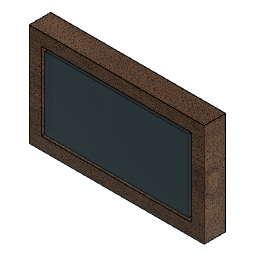
Glowing Square (Autodesk Fusion 360 design; units mm, degrees)
Autodesk Fusion 360 part; units mm, degrees
sketch "Sketch2" plane through (0, 0, 0) normal (0, 1, 0) x (1, 0, 0)
  line L0 (0, 0) -> (256, 0)
  line L1 (256, 0) -> (256, 128)
  line L2 (256, 128) -> (0, 128)
  line L3 (0, 128) -> (0, 0)
  dimension "d1" = 256
  dimension "d2" = 128
  constraint horizontal L0
  constraint vertical L1
  constraint horizontal L2
  constraint vertical L3
  constraint coincident L0.start L3.end
  measures "d1" distance of L0.start L0.end
  measures "d2" distance of L0.start L2.end
extrude "Extrude1" add sketch "Sketch2" along normal blind 14 makes body 1
chamfer "Chamfer1" distance 1 distance2 14 4 edges at (128, 14, 0) (256, 14, -64) (0, 14, -64) (128, 14, -128) measured on face at (85.3333, 14, -85.3333) measured on face at (85.3333, 14, -85.3333) measured on face at (85.3333, 14, -85.3333) measured on face at (85.3333, 14, -85.3333) on bodies 1
sketch "Sketch3" plane through (0, 14, 0) normal (0, 1, 0) x (-1, 0, 0)
  line L0 (-255, -127) -> (-1, -127)
  line L1 (-1, -127) -> (-1, -1)
  line L2 (-1, -1) -> (-255, -1)
  line L3 (-255, -1) -> (-255, -127)
  circle A0 centre (-248, -8) radius 1.5
  circle A1 centre (-128, -8) radius 1.5
  circle A2 centre (-8, -8) radius 1.5
  circle A3 centre (-248, -120) radius 1.5
  circle A4 centre (-128, -120) radius 1.5
  circle A5 centre (-8, -120) radius 1.5
  dimension "d7" = 3
  dimension "d8" = 7
  dimension "d9" = 7
  dimension "d10" = 3
  dimension "d11" = 127
  dimension "d12" = 3
  dimension "d13" = 7
  dimension "d14" = 3
  dimension "d15" = 7
  dimension "d16" = 3
  dimension "d17" = 3
  measures "d7" diameter of A0
  measures "d8" distance of L3 A0.centre
  measures "d9" distance of L2 A0.centre
  measures "d10" diameter of A1
  measures "d11" distance of L3 A1.centre
  measures "d12" diameter of A2
  measures "d13" distance of L1 A2.centre
  measures "d14" diameter of A3
  measures "d15" distance of L0 A3.centre
  measures "d16" diameter of A4
  measures "d17" diameter of A5
extrude "Extrude2" cut sketch "Sketch3" against normal blind 10 contours A0 | A1 | A2 | A3 | A4 | A5 bodies 1
sketch "Sketch4" plane through (0, 14, 0) normal (0, 1, 0) x (-1, 0, 0)
  circle A0 centre (-8, -120) radius 1.5
  circle A1 centre (-248, -8) radius 1.5
  circle A2 centre (-128, -120) radius 1.5
  circle A3 centre (-8, -8) radius 1.5
  circle A4 centre (-128, -8) radius 1.5
  circle A5 centre (-248, -120) radius 1.5
  line L0 (-255, -127) -> (-1, -127)
  line L1 (-1, -127) -> (-1, -1)
  line L2 (-1, -1) -> (-255, -1)
  line L3 (-255, -1) -> (-255, -127)
  line L4 (-103, -24) -> (-43, -24)
  line L5 (-43, -24) -> (-43, -104)
  line L6 (-43, -104) -> (-103, -104)
  line L7 (-103, -104) -> (-103, -24)
  dimension "d20" = 60
  dimension "d21" = 80
  dimension "d22" = 42
  dimension "d23" = 23
  constraint horizontal L4
  constraint vertical L5
  constraint horizontal L6
  constraint vertical L7
  measures "d20" distance of L4.start L4.end
  measures "d21" distance of L4.start L6.end
  measures "d22" distance of L1 L5
  measures "d23" distance of L0 L6
extrude "Extrude3" add sketch "Sketch4" along normal blind 20 contours L4 L5 L6 L7 bodies 1
sketch "Sketch5" plane through (0, 0, 0) normal (0, -1, 0) x (1, 0, 0)
  line L0 (0, 0) -> (0, -128)
  line L1 (0, -128) -> (256, -128)
  line L2 (256, -128) -> (256, 0)
  line L3 (256, 0) -> (0, 0)
copy_body "CutPasteBodies1" bodies 1 removing the originals makes body 2 in component "Display"
sketch "Sketch1" plane through (0, 14, 0) normal (0, 1, 0) x (-1, 0, 0) in component "Display"
  line L0 (-103, -104) -> (-103, -24)
  line L1 (-103, -24) -> (-43, -24)
  line L2 (-43, -24) -> (-43, -104)
  line L3 (-43, -104) -> (-103, -104)
  circle A0 centre (-8, -120) radius 1.5
  circle A1 centre (-248, -8) radius 1.5
  circle A2 centre (-128, -120) radius 1.5
  circle A3 centre (-8, -8) radius 1.5
  circle A4 centre (-128, -8) radius 1.5
  circle A5 centre (-248, -120) radius 1.5
  line L4 (-255, -127) -> (-1, -127)
  line L5 (-1, -127) -> (-1, -1)
  line L6 (-1, -1) -> (-255, -1)
  line L7 (-255, -1) -> (-255, -127)
sketch "Sketch1 (2)" plane through (0, 0, 0) normal (0, 1, 0) x (1, 0, 0) in component "Frame"
  line L0 (-27, -27) -> (283, -27)
  line L1 (283, -27) -> (283, 155)
  line L2 (283, 155) -> (-27, 155)
  line L3 (-27, 155) -> (-27, -27)
  line L4 (-5, -5) -> (261, -5)
  line L5 (261, -5) -> (261, 133)
  line L6 (261, 133) -> (-5, 133)
  line L7 (-5, 133) -> (-5, -5)
  dimension "d26" = 310
  dimension "d27" = 182
  dimension "d28" = 27
  dimension "d29" = 27
  dimension "d30" = 22
  dimension "d31" = 22
  dimension "d32" = 22
  dimension "d33" = 22
  constraint horizontal L0
  constraint vertical L1
  constraint horizontal L2
  constraint vertical L3
  constraint horizontal L4
  constraint vertical L5
  constraint horizontal L6
  constraint vertical L7
  measures "d26" distance of L0.start L0.end
  measures "d27" distance of L0.start L2.end
  measures "d28" distance of origin L3
  measures "d29" distance of L0 origin
  measures "d30" distance of L3 L7
  measures "d31" distance of L1 L5
  measures "d32" distance of L0 L4
  measures "d33" distance of L2 L6
extrude "Extrude1'" add sketch "Sketch1 (2)" along normal blind 38 separate body makes body 3 in component "Frame"
sketch "Sketch1 (3)" plane through (0, 14, 0) normal (0, 1, 0) x (-1, 0, 0) in component "Display Mount"
  line L0 (-103, -104) -> (-103, -24)
  line L1 (-103, -24) -> (-43, -24)
  line L2 (-43, -24) -> (-43, -104)
  line L3 (-43, -104) -> (-103, -104)
  circle A0 centre (-8, -120) radius 1.5
  circle A1 centre (-248, -8) radius 1.5
  circle A2 centre (-128, -120) radius 1.5
  circle A3 centre (-8, -8) radius 1.5
  circle A4 centre (-128, -8) radius 1.5
  circle A5 centre (-248, -120) radius 1.5
  line L4 (-255, -127) -> (-1, -127)
  line L5 (-1, -127) -> (-1, -1)
  line L6 (-1, -1) -> (-255, -1)
  line L7 (-255, -1) -> (-255, -127)
  line L8 (-261, 5) -> (5, 5)
  line L9 (5, 5) -> (5, -133)
  line L10 (5, -133) -> (-261, -133)
  line L11 (-261, -133) -> (-261, 5)
  line L12 (-256, -128) -> (-256, 0)
  line L13 (-256, 0) -> (0, 0)
  line L14 (-243, -13) -> (-13, -13)
  line L15 (-13, -13) -> (-13, -115)
  line L16 (-13, -115) -> (-243, -115)
  line L17 (-243, -115) -> (-243, -13)
  dimension "d36" = 266
  dimension "d37" = 138
  dimension "d38" = 5
  dimension "d39" = 5
  dimension "d40" = 5
  dimension "d41" = 5
  dimension "d42" = 5
  dimension "d43" = 5
  constraint horizontal L8
  constraint vertical L9
  constraint horizontal L10
  constraint vertical L11
  constraint horizontal L14
  constraint vertical L15
  constraint horizontal L16
  constraint vertical L17
  measures "d36" distance of L8.start L8.end
  measures "d37" distance of L8.start L10.end
  measures "d38" distance of L11 L12
  measures "d39" distance of L8 L13
  measures "d40" distance of A1.centre L17
  measures "d41" distance of A1.centre L14
  measures "d42" distance of A3.centre L15
  measures "d43" distance of A0.centre L16
extrude "Extrude1''" add sketch "Sketch1 (3)" along normal blind 4 separate body contours L4 L5 L6 L7 | L8 L9 L10 L11 makes body 4 in component "Display Mount"
sketch "Sketch2 (2)" plane through (0, 18, 0) normal (0, 1, 0) x (-1, 0, 0) in component "Display Mount"
  circle A0 centre (-8, -8) radius 1.5
  circle A1 centre (-128, -8) radius 1.5
  circle A2 centre (-248, -120) radius 1.5
  circle A3 centre (-8, -120) radius 1.5
  circle A4 centre (-248, -8) radius 1.5
  line L0 (-13, -115) -> (-243, -115)
  line L1 (-243, -115) -> (-243, -13)
  line L2 (-243, -13) -> (-13, -13)
  line L3 (-13, -13) -> (-13, -115)
  circle A5 centre (-128, -120) radius 1.5
  line L4 (-261, -133) -> (5, -133)
  line L5 (5, -133) -> (5, 5)
  line L6 (5, 5) -> (-261, 5)
  line L7 (-261, 5) -> (-261, -133)
  line L8 (-231, 5) -> (-216, 5)
  line L9 (-216, 5) -> (-216, -1)
  line L10 (-216, -1) -> (-231, -1)
  line L11 (-231, -1) -> (-231, 5)
  line L12 (-40, 5) -> (-25, 5)
  line L13 (-25, 5) -> (-25, -1)
  line L14 (-25, -1) -> (-40, -1)
  line L15 (-40, -1) -> (-40, 5)
  line L16 (-261, -55.5) -> (-255, -55.5)
  line L17 (-255, -55.5) -> (-255, -70.5)
  line L18 (-255, -70.5) -> (-261, -70.5)
  line L19 (-261, -70.5) -> (-261, -55.5)
  line L20 (-231, -133) -> (-216, -133)
  line L21 (-216, -133) -> (-216, -127)
  line L22 (-216, -127) -> (-231, -127)
  line L23 (-231, -127) -> (-231, -133)
  line L24 (5, -55.5) -> (-1, -55.5)
  line L25 (-1, -55.5) -> (-1, -70.5)
  line L26 (-1, -70.5) -> (5, -70.5)
  line L27 (5, -70.5) -> (5, -55.5)
  line L28 (-40, -133) -> (-25, -133)
  line L29 (-25, -133) -> (-25, -127)
  line L30 (-25, -127) -> (-40, -127)
  line L31 (-40, -127) -> (-40, -133)
  dimension "d46" = 15
  dimension "d47" = 6
  dimension "d48" = 30
  dimension "d49" = 15
  dimension "d50" = 6
  dimension "d51" = 30
  dimension "d52" = 6
  dimension "d53" = 15
  dimension "d54" = 60.5
  dimension "d55" = 15
  dimension "d56" = 6
  dimension "d57" = 30
  dimension "d58" = 6
  dimension "d59" = 15
  dimension "d60" = 60.5
  dimension "d61" = 15
  dimension "d62" = 6
  dimension "d63" = 30
  constraint horizontal L8
  constraint vertical L9
  constraint horizontal L10
  constraint vertical L11
  constraint coincident L6 L8.start
  constraint horizontal L12
  constraint vertical L13
  constraint horizontal L14
  constraint vertical L15
  constraint coincident L6 L12.start
  constraint horizontal L16
  constraint vertical L17
  constraint horizontal L18
  constraint vertical L19
  constraint coincident L7 L16.start
  constraint horizontal L20
  constraint vertical L21
  constraint horizontal L22
  constraint vertical L23
  constraint coincident L4 L20.start
  constraint horizontal L24
  constraint vertical L25
  constraint horizontal L26
  constraint vertical L27
  constraint coincident L5 L24.start
  constraint horizontal L28
  constraint vertical L29
  constraint horizontal L30
  constraint vertical L31
  constraint coincident L4 L28.start
  measures "d46" distance of L8.start L8.end
  measures "d47" distance of L8.start L10.end
  measures "d48" distance of L7 L11
  measures "d49" distance of L12.start L12.end
  measures "d50" distance of L12.start L14.end
  measures "d51" distance of L5 L13
  measures "d52" distance of L16.start L16.end
  measures "d53" distance of L16.start L18.end
  measures "d54" distance of L6 L16
  measures "d55" distance of L20.start L20.end
  measures "d56" distance of L20.start L22.end
  measures "d57" distance of L7 L23
  measures "d58" distance of L24.start L24.end
  measures "d59" distance of L24.start L26.end
  measures "d60" distance of L6 L24
  measures "d61" distance of L28.start L28.end
  measures "d62" distance of L28.start L30.end
  measures "d63" distance of L5 L29
extrude "Extrude2'" add sketch "Sketch2 (2)" along normal blind 12 contours L4 L20 L21 L22 L23 | L7 L16 L17 L18 L19 | L4 L28 L29 L30 L31 | L6 L8 L9 L10 L11 | L5 L24 L25 L26 L27 | L6 L12 L13 L14 L15 bodies 4 in component "Display Mount"
fillet "Fillet1" radius 2 18 edges at (216, 18, 2) (25, 18, 2) (231, 18, 2) (40, 18, 2) (-2, 18, -70.5) (-2, 18, -55.5) (223.5, 18, -1) (32.5, 18, -1) (255, 18, -63) (258, 18, -70.5) (1, 18, -63) (32.5, 18, -127) (40, 18, -130) (223.5, 18, -127) (216, 18, -130) (258, 18, -55.5) (25, 18, -130) (231, 18, -130) on bodies 4 in component "Display Mount"
hole "Hole1" at (32.5, 25, -1) direction (0, 0, 1) diameter 4 depth 6 tip angle 180 countersink diameter 6.6 countersink angle 90 bodies 4 in component "Display Mount"
hole "Hole2" at (223.5, 25, -1) direction (0, 0, 1) diameter 4 depth 6 tip angle 180 countersink diameter 6.6 countersink angle 90 bodies 4 in component "Display Mount"
hole "Hole3" at (255, 25, -63) direction (1, 0, 0) diameter 4 depth 6 tip angle 180 countersink diameter 6.6 countersink angle 90 bodies 4 in component "Display Mount"
hole "Hole4" at (223.5, 25, -127) direction (0, 0, -1) diameter 4 depth 6 tip angle 180 countersink diameter 6.6 countersink angle 90 bodies 4 in component "Display Mount"
hole "Hole5" at (32.5, 25, -127) direction (0, 0, -1) diameter 4 depth 6 tip angle 180 countersink diameter 6.6 countersink angle 90 bodies 4 in component "Display Mount"
hole "Hole6" at (1, 25, -63) direction (-1, 0, 0) diameter 4 depth 6 tip angle 180 countersink diameter 6.6 countersink angle 90 bodies 4 in component "Display Mount"
sketch "Sketch1 (4)" plane through (0, 38, 0) normal (0, 1, 0) x (-1, 0, 0) in component "Wall Mount"
  line L0 (5, 5) -> (5, -133)
  line L1 (5, -133) -> (-261, -133)
  line L2 (-261, -133) -> (-261, 5)
  line L3 (-261, 5) -> (5, 5)
  line L4 (27, -155) -> (27, 27)
  line L5 (27, 27) -> (-283, 27)
  line L6 (-283, 27) -> (-283, -155)
  line L7 (-283, -155) -> (27, -155)
  line L8 (-271, 15) -> (15, 15)
  line L9 (15, 15) -> (15, -143)
  line L10 (15, -143) -> (-271, -143)
  line L11 (-271, -143) -> (-271, 15)
  dimension "d97" = 286
  dimension "d98" = 158
  dimension "d99" = 10
  dimension "d100" = 10
  constraint horizontal L8
  constraint vertical L9
  constraint horizontal L10
  constraint vertical L11
  measures "d97" distance of L8.start L8.end
  measures "d98" distance of L8.start L10.end
  measures "d99" distance of L3 L8
  measures "d100" distance of L2 L11
extrude "Extrude1'''" add sketch "Sketch1 (4)" along normal blind 2 separate body contours L0 L1 L2 L3 | L8 L9 L10 L11 makes body 5 in component "Wall Mount"
sketch "Sketch2 (3)" plane through (0, 0, -155) normal (0, 0, -1) x (1, 0, 0) in component "Frame"
  line L0 (283, 0) -> (-27, 0)
  line L1 (-27, 0) -> (-27, -38)
  line L2 (-27, -38) -> (283, -38)
  line L3 (283, -38) -> (283, 0)
sketch "Sketch3 (2)" plane through (0, 0, -155) normal (0, 0, -1) x (1, 0, 0) in component "Frame"
  circle A0 centre (128, -34) radius 4
  line L0 (-27, 0) -> (-27, -38)
  line L1 (-27, -38) -> (283, -38)
  line L2 (132, -38) -> (124, -38)
  line L3 (124, -38) -> (124, -34)
  line L4 (124, -34) -> (132, -34)
  line L5 (132, -34) -> (132, -38)
  dimension "d106" = 8
  dimension "d107" = 155
  dimension "d108" = 4
  dimension "d109" = 8
  constraint horizontal L2
  constraint vertical L3
  constraint horizontal L4
  constraint vertical L5
  constraint coincident A0 L3.end
  constraint coincident L1 L2.start
  measures "d106" diameter of A0
  measures "d107" distance of A0.centre L0
  measures "d108" distance of A0.centre L1
  measures "d109" distance of L3.end L4.end
extrude "Extrude2''" cut sketch "Sketch3 (2)" against normal blind 22 bodies 3 in component "Frame"
sketch "Sketch3 (3)" plane through (0, 38, 0) normal (0, -1, 0) x (1, 0, 0) in component "Wall Mount"
  line L0 (-15, -143) -> (271, -143)
  line L1 (271, -143) -> (271, 15)
  line L2 (271, 15) -> (-15, 15)
  line L3 (-15, 15) -> (-15, -143)
  line L4 (-5, 5) -> (261, 5)
  line L5 (261, 5) -> (261, -133)
  line L6 (261, -133) -> (-5, -133)
  line L7 (-5, -133) -> (-5, 5)
  dimension "d140" = 266
  dimension "d141" = 138
  dimension "d142" = 10
  dimension "d143" = 10
  constraint horizontal L4
  constraint vertical L5
  constraint horizontal L6
  constraint vertical L7
  measures "d140" distance of L4.start L4.end
  measures "d141" distance of L4.start L6.end
  measures "d142" distance of L2 L4
  measures "d143" distance of L3 L7
extrude "Extrude3'" add sketch "Sketch3 (3)" along normal blind 2 contours L4 L5 L6 L7 bodies 5 in component "Wall Mount"
sketch "Sketch2 (4)" plane through (0, 40, 0) normal (0, 1, 0) x (-1, 0, 0) in component "Wall Mount"
  line L0 (-271, -143) -> (15, -143)
  line L1 (15, -143) -> (15, 15)
  line L2 (15, 15) -> (-271, 15)
  line L3 (-271, 15) -> (-271, -143)
  circle A0 centre (-266, 10) radius 2
  circle A1 centre (10, 10) radius 2
  circle A2 centre (-266, -138) radius 2
  circle A3 centre (10, -138) radius 2
  circle A4 centre (-128, -25) radius 7
  circle A5 centre (-128, -18) radius 3.5
  dimension "d112" = 4
  dimension "d113" = 5
  dimension "d114" = 5
  dimension "d115" = 4
  dimension "d116" = 5
  dimension "d117" = 5
  dimension "d118" = 4
  dimension "d119" = 5
  dimension "d120" = 5
  dimension "d121" = 4
  dimension "d122" = 5
  dimension "d123" = 5
  dimension "d134" = 14
  dimension "d135" = 143
  dimension "d136" = 40
  dimension "d146" = 7
  constraint coincident A4 A5.centre
  measures "d112" diameter of A0
  measures "d113" distance of L2 A0.centre
  measures "d114" distance of L3 A0.centre
  measures "d115" diameter of A1
  measures "d116" distance of L1 A1.centre
  measures "d117" distance of L2 A1.centre
  measures "d118" diameter of A2
  measures "d119" distance of L0 A2.centre
  measures "d120" distance of L3 A2.centre
  measures "d121" diameter of A3
  measures "d122" distance of L1 A3.centre
  measures "d123" distance of L0 A3.centre
  measures "d134" diameter of A4
  measures "d135" distance of L3 A4.centre
  measures "d136" distance of L2 A4.centre
  measures "d146" diameter of A5
extrude "Extrude2'''" cut sketch "Sketch2 (4)" against normal blind 10 contours A4 A5 | A4 A5 | A4 A5 bodies 5 in component "Wall Mount"
hole "Hole2'" [suppressed] in component "Frame"
hole "Hole1'" at (266, 40, 10) at (-10, 40, 10) at (-10, 40, -138) at (266, 40, -138) direction (0, -1, 0) diameter 4 depth 2 tip angle 180 countersink diameter 6.6 countersink angle 90 bodies 5 in component "Wall Mount"
component "Display" placed x (1, 0, 0) y (0, 1, 0) z (0, 0, 1) at (0, 0, 0)
component "Frame" placed x (1, 0, 0) y (0, 1, 0) z (0, 0, 1) at (0, 0, 0)
component "Display Mount" placed x (1, 0, 0) y (0, 1, 0) z (0, 0, 1) at (0, 0, 0) in component "Display"
component "Wall Mount" placed x (1, 0, 0) y (0, 1, 0) z (0, 0, 1) at (0, 0, 0) in component "Frame"
equation "d28 = 32 mm - 5 mm"
equation "d29 = 32 mm - 5 mm"
equation "d49 = d46"
equation "d51 = d48"
equation "d53 = d46"
equation "d54 = ( ( 136 / 2 ) * 1 mm ) - d46 / 2"
equation "d55 = d46"
equation "d57 = d48"
equation "d59 = d46"
equation "d60 = d54"
equation "d61 = d46"
equation "d63 = d51"
equation "d97 = 256 mm + 30 mm"
equation "d98 = 128 mm + 30 mm"
equation "d107 = ( ( 256 + 10 + 44 ) / 2 ) * 1 mm"
equation "d113 = d114"
equation "d116 = d114"
equation "d117 = d114"
equation "d119 = d114"
equation "d120 = d114"
equation "d122 = d114"
equation "d123 = d114"
equation "d135 = ( 286 / 2 ) * 1 mm"
equation "d140 = 286 mm - 20 mm"
